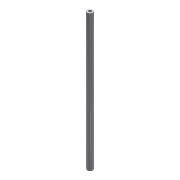
# Autodesk Inventor part: Barra-garfo
Saved by Autodesk Inventor 2015 (Build 190159000, 159)
## iProperties
Created: 2016-08-11
Part Number: Barra-garfo
Material: Aluminium AW-7020
Document SubType Name: Modeling
Designer: EriveltonDell
Density: 2.78 g/cm^3
Appearance: Aluminum - Dark
Mass: 323.166 g
Surface Area: 250.401 cm^2
Volume: 116.247 cm^3
Author: EriveltonDell
Autodesk Inventor part; units mm, degrees
ref_plane "YZ Plane" through (0, 0, 0) normal (1, 0, 0) x (0, 1, 0)
ref_plane "XZ Plane" through (0, 0, 0) normal (0, 1, 0) x (-1, 0, 0)
ref_plane "XY Plane" through (0, 0, 0) normal (0, 0, 1) x (1, 0, 0)
sketch "Sketch1" plane through (0, 0, 0) normal (0, 0, 1) x (1, 0, 0)
  circle A0 centre (0, 0) radius 9.5
  dimension "d0" = 19
  constraints: 1 centre point, 1 coincident
  measures "d0" diameter of A0
extrude "Extrusion1" add sketch "Sketch1" along normal blind 470
hole "Hole1" at (0, 0, 470) direction (0, 0, -1) diameter 10 depth 70 tip angle 118
hole "Hole2" at (0, 0, 0) direction (0, 0, 1) diameter 10 depth 70 tip angle 118
body "Solid1"
